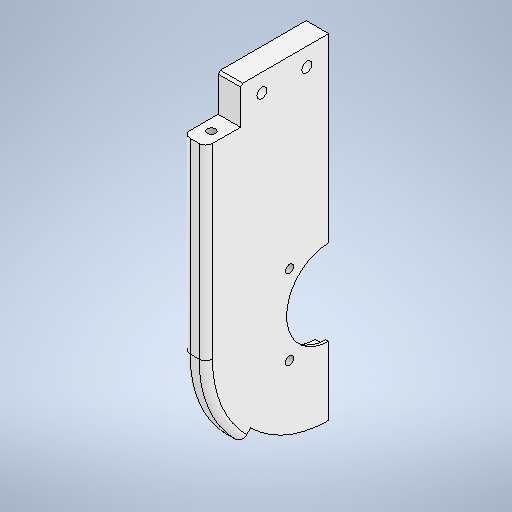
# Autodesk Inventor part: joint3_frame_support1
Saved by Autodesk Inventor 2025.3 (Build 293356030, 356C)
## iProperties
Created: 2025-11-25
Part Number: joint3_frame_support1
Material: PLA filament
Document SubType Name: Modeling
Designer: MSI
Density: 1.2 g/cm^3
Appearance: 일반
Mass: 75.1328 g
Surface Area: 185.308 cm^2
Volume: 62.6107 cm^3
Author: MSI
Autodesk Inventor part; units mm, degrees
ref_plane "YZ Plane" through (0, 0, 0) normal (1, 0, 0) x (0, 1, 0)
ref_plane "XZ Plane" through (0, 0, 0) normal (0, 1, 0) x (-1, 0, 0)
sketch "스케치1" plane through (0, 0, 0) normal (1, 0, 0) x (0, 1, 0)
  circle A0 centre (0, 0) radius 55
  line L0 (0, 55) -> (99.7, 55)
  line L1 (99.7, 55) -> (99.7, -55)
  line L2 (99.7, -55) -> (0, -55)
  line L3 (0, -55) -> (0, 55)
  dimension "d0" = 110
  dimension "d1" = 99.7
  constraints: 8 end point, 2 parallel, 2 point on circle, 1 centre point, 1 coincident, 1 horizontal, 1 midpoint, 1 perpendicular
  measures "d0" diameter of A0
  measures "d1" distance of L1.end L2.end
extrude "돌출1" add sketch "스케치1" along normal mid plane 10
sketch "스케치5" plane through (-5, 0, 0) normal (-1, 0, 0) x (0, 0, 1)
  line L0 (-55, 99.7) -> (55, 99.7) projected
  line L1 (-55, 99.7) -> (-39.5, 99.7)
  line L2 (-39.5, 99.7) -> (-39.5, 83.2)
  line L3 (-39.5, 83.2) -> (-55, 83.2)
  line L4 (-55, 83.2) -> (-55, 99.7)
  line L5 (55, 99.7) -> (39.5, 99.7)
  line L6 (39.5, 99.7) -> (39.5, 83.2)
  line L7 (39.5, 83.2) -> (55, 83.2)
  line L8 (55, 83.2) -> (55, 99.7)
  point P0 (0, 0)
  dimension "d31" = 16.5
  dimension "d32" = 15.5
  dimension "d33" = 15.5
  constraints: 16 end point, 4 parallel, 2 horizontal, 2 perpendicular, 1 point on line
  measures "d31" distance of L3.end L0.start
  measures "d32" distance of L2.end L3.end
  measures "d33" distance of L6.end L7.end
extrude "돌출2" cut sketch "스케치5" against normal through all
sketch "스케치2" plane through (-5, 0, 0) normal (-1, 0, 0) x (0, 0, 1)
  arc A0 (-55, 0) -> (55, 0) centre (0, 0) ccw projected
  constraints: 1 coincident
hole "구멍1" at (-5, 0, 0) direction (1, 0, 0) diameter 38 end through all counterbore diameter 42.5 counterbore depth 8.75
sketch "스케치3" plane through (-5, 0, 0) normal (-1, 0, 0) x (0, 0, 1)
  circle A0 centre (0, 0) radius 21.25 projected
  constraints: 1 coincident
hole "구멍2" at (-5, 0, 0) direction (1, 0, 0) diameter 58.5 depth 3
sketch "스케치4" plane through (-2, 0, 0) normal (-1, 0, 0) x (0, 0, 1)
  line L0 (0, 0) -> (17.6777, 17.6777)
  line L1 (0, 0) -> (25, 0) construction
  dimension "d19" = 25
  dimension "d20" = 45
  constraints: 4 end point, 1 equal length, 1 horizontal
  measures "d19" distance of L0.start L0.end
  measures "d20" angle of L1 L0
hole "구멍3" at (-2, 17.6777, 17.6777) direction (1, 0, 0) diameter 3.6881 end through all thread size "M4.5x0.75" class "6H" standard "ISO Metric profile"
pattern_circular "원형 패턴1" count 4 over 360 about axis through (-0.625, 0, 0) along (-1, 0, 0) of "구멍3"
sketch "스케치6" plane through (-5, 0, 0) normal (-1, 0, 0) x (0, 0, 1)
  line L0 (-30, 91.7) -> (30, 91.7) construction
  line L1 (39.5, 99.7) -> (-39.5, 99.7) projected
  point P0 (0, 0)
  point P1 (0, 91.7)
  point P2 (0, 99.7)
  point P3 (-10, 91.7)
  point P4 (10, 91.7)
  dimension "d40" = 8
  dimension "d41" = 20
  dimension "d42" = 20
  dimension "d43" = 60
  constraints: 2 coincident, 2 end point, 2 midpoint, 2 point on line, 1 horizontal, 1 vertical alignment
  measures "d40" distance between parallel lines of L0 L1
  measures "d41" distance of point (-10, 91.7) L0.start
  measures "d42" distance of L0.end point (10, 91.7)
  measures "d43" distance of L0.start L0.end
hole "구멍4" at (-5, 91.7, -30) at (-5, 91.7, 30) at (-5, 91.7, -10) at (-5, 91.7, 10) direction (1, 0, 0) diameter 4.5 end through all counterbore diameter 8 counterbore depth 4.6 clearance for "Socket Head Cap Screw ISO 4762" size "M4" standard "ISO"
sketch "스케치7" plane through (-5, 83.2, 55) normal (0, 1, 0) x (1, 0, 0)
  line L0 (5, 102.5) -> (5, 7.5) construction
  line L1 (0, 110) -> (10, 110) projected
  point P0 (5, 55)
  point P1 (5, 55)
  dimension "d51" = 7.5
  constraints: 3 coincident, 2 end point, 1 midpoint, 1 vertical
  measures "d51" distance from line of point (5, 102.5) L1
hole "구멍5" at (0, 83.2, -47.5) at (0, 83.2, 47.5) direction (0, -1, 0) diameter 3.6881 depth 13 tip angle 118 thread size "M4.5x0.75" class "6H" standard "ISO Metric profile"
fillet "모깎기1" radius 3 6 edges at (5, -55, 0) (5, 41.6, -55) (5, 41.6, 55) (-5, -55, 0) (-5, 41.6, -55) (-5, 41.6, 55)
chamfer "모따기1" distance 1 angle 45 3 edges at (0, 99.7, -39.5) (0, 99.7, 39.5) (-2, 0, -21.25)
fillet "모깎기2" radius 0.1 1 edges at (3.75, 0, -21.25)
sketch "스케치8" plane through (0, 0, 0) normal (1, 0, 0) x (0, 1, 0)
  arc A0 (0, 55) -> (0, -55) centre (0, 0) ccw projected
  line L0 (-38.8909, 38.8909) -> (0, 0)
  line L1 (0, 0) -> (-55, 0)
  arc A1 (0, 49.5) -> (0, -49.5) centre (0, 0) ccw
  point P0 (-49.5, 0)
  point P1 (-35.0018, 35.0018)
  dimension "d59" = 45
  dimension "d60" = 5.5
  constraints: 4 end point, 4 point on circle, 1 centre point
  measures "d59" angle of L1 L0
  measures "d60" radial gap between concentric circles of A0 A1
extrude "돌출3" cut sketch "스케치8" along normal through all both and the other way through all contours L0 A1 L1 A0
sketch "스케치9" plane through (0, 0, 0) normal (1, 0, 0) x (0, 1, 0)
  line L0 (0, 0) -> (-40.548, 28.392) construction
  arc A0 (-35.0018, 35.0018) -> (-49.5, 0) centre (0, 0) ccw construction
  line L1 (0, 0) -> (-49.5, 0) construction
  dimension "d63" = 35
  constraints: 4 end point, 1 horizontal, 1 point on circle
  measures "d63" angle of L1 L0
ref_plane "작업 평면1" through (0, -40.548, 28.392) normal (0, -0.819152, 0.5735764) x (1, 0, 0)
sketch "스케치10" plane through (0, -40.548, 28.392) normal (0, -0.819152, 0.5735764) x (1, 0, 0)
  point P0 (0, 0)
  point P1 (0, 0)
  constraints: 1 coincident
hole "구멍6" at (0, -40.548, 28.392) direction (0, 0.819152, -0.5735764) diameter 3.6881 depth 13 tip angle 118 thread size "M4.5x0.75" class "6H" standard "ISO Metric profile"
mirror "미러1" about plane through (0, 0, 0) normal (0, 0, 1) of "구멍6", "돌출3"
sketch "스케치11" plane through (5, 0, 0) normal (1, 0, 0) x (0, 0, -1)
  line L0 (-0.25, 113.4459) -> (-97.7247, 113.4459)
  line L1 (-97.7247, 113.4459) -> (-97.7247, -72.0948)
  line L2 (-97.7247, -72.0948) -> (-0.25, -72.0948)
  line L3 (-0.25, -72.0948) -> (-0.25, 113.4459)
  point P0 (0, 0)
  dimension "d71" = 0.25
  constraints: 8 end point, 2 parallel, 1 horizontal, 1 perpendicular
  measures "d71" distance from line of point (0, 0) L3
extrude "돌출4" cut sketch "스케치11" against normal through all keep common part
sketch "스케치12" plane through (5, 18.9984, 0.25) normal (0, 0, -1) x (-1, 0, 0)
  line L0 (5, 51.0016) -> (5, -53.9984) construction
  point P0 (5, -18.9984)
  point P1 (5, 16.0016)
  dimension "d77" = 35
  dimension "d78" = 35
  dimension "d80" = 105
  constraints: 2 coincident, 2 end point, 2 point on line, 1 vertical
  measures "d77" distance of point (5, -18.998) point (5, -53.998)
  measures "d78" distance of point (5, 16.002) point (5, -18.998)
  measures "d80" distance of L0.start L0.end
hole "구멍7" at (0, 70, 0.25) at (0, 35, 0.25) at (0, -35, 0.25) direction (0, 0, 1) diameter 4.5 depth 10 tip angle 118
equation "\"d33\" = d32"
equation "\"d42\" = d41"
equation "\"d43\" = 3 * d41"
equation "\"d78\" = d77"
equation "\"d80\" = 3 * d77"
